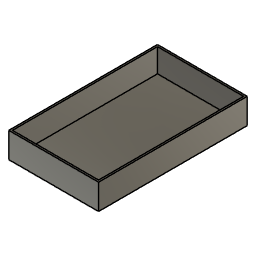
Full+Casing (Autodesk Fusion 360 design; units mm, degrees)
Autodesk Fusion 360 part; units mm, degrees
sketch "Sketch1" plane through (0, 0, 0) normal (0, 0, 1) x (1, 0, 0)
  line L0 (47.5, 80) -> (-47.5, 80)
  line L1 (-47.5, 80) -> (-47.5, -80)
  line L2 (-47.5, -80) -> (47.5, -80)
  line L3 (47.5, -80) -> (47.5, 80)
  line L4 (47.5, 80) -> (-47.5, -80) construction
  line L5 (-47.5, 80) -> (47.5, -80) construction
  line L6 (-49.5, -82) -> (49.5, -82)
  line L7 (49.5, -82) -> (49.5, 82)
  line L8 (49.5, 82) -> (-49.5, 82)
  line L9 (-49.5, 82) -> (-49.5, -82)
  dimension "d1" = 95
  dimension "d2" = 160
  dimension "d3" = 2
  constraint horizontal L0
  constraint perpendicular L0 L1
  constraint parallel L0 L2
  constraint parallel L1 L3
  constraint coincident L4 origin
  constraint coincident L5 origin
  measures "d1" distance of L1.end L2.end
  measures "d2" distance of L0.end L1.end
extrude "Extrude1" add sketch "Sketch1" along normal blind 28 makes body 1
sketch "Sketch2" plane through (0, 0, 0) normal (0, 0, 1) x (1, 0, 0)
  line L0 (47.5, 80) -> (47.5, -80)
  line L1 (47.5, 80) -> (47.5, -80)
  line L2 (47.5, -80) -> (-47.5, -80)
  line L3 (-47.5, -80) -> (-47.5, 80)
  line L4 (-47.5, 80) -> (47.5, 80)
  line L5 (-49.5, 82) -> (-49.5, -82)
  line L6 (-49.5, -82) -> (49.5, -82)
  line L7 (49.5, -82) -> (49.5, 82)
  line L8 (49.5, 82) -> (-49.5, 82)
  line L9 (-47.5, 80) -> (47.5, 80)
  line L10 (47.5, 80) -> (47.5, -80)
  line L11 (47.5, -80) -> (-47.5, -80)
  line L12 (-47.5, -80) -> (-47.5, 80)
  constraint horizontal L9
  constraint vertical L10
  constraint horizontal L11
  constraint vertical L12
  constraint coincident L0.end L1.end
  constraint coincident L3.end L4.start
extrude "Extrude2" add sketch "Sketch2" along normal blind 2 contours L0 L1 L2 L3 L4 L9 L10 L11 L12 bodies 1
copy_body "Body->Comp1" bodies 1 removing the originals makes body 2 in component "Bottom Case"
sketch "Sketch3" plane through (0, 0, 28) normal (0, 0, 1) x (-1, 0, 0)
  line L0 (-47.5, -80) -> (-47.5, 80)
  line L1 (-47.5, 80) -> (47.5, 80)
  line L2 (47.5, 80) -> (47.5, -80)
  line L3 (47.5, -80) -> (-47.5, -80)
  line L4 (49.5, -82) -> (49.5, 82)
  line L5 (49.5, 82) -> (-49.5, 82)
  line L6 (-49.5, 82) -> (-49.5, -82)
  line L7 (-49.5, -82) -> (49.5, -82)
  line L8 (-49.5, 82) -> (49.5, 82)
  line L9 (49.5, 82) -> (49.5, -82)
  line L10 (49.5, -82) -> (-49.5, -82)
  line L11 (-49.5, -82) -> (-49.5, 82)
  constraint horizontal L8
  constraint vertical L9
  constraint horizontal L10
  constraint vertical L11
  constraint coincident L4.start L7.end
  constraint coincident L5.end L6.start
extrude "Extrude1'" add sketch "Sketch3" along normal blind 2 separate body contours L0 L1 L2 L3 | L4 L5 L6 L7 L8 L9 L10 L11 makes body 3 in component "Top Case"
component "Bottom Case" placed x (1, 0, 0) y (0, 1, 0) z (0, 0, 1) at (0, 0, 0)
component "Top Case" placed x (1, 0, 0) y (0, 1, 0) z (0, 0, 1) at (0, 0, 0)
equation "d4 = 30 mm - 2 mm"
